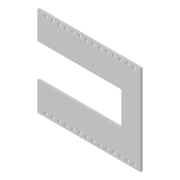
# Autodesk Inventor part: Flat Roof panel
Saved by Autodesk Inventor 2018 (Build 220112000, 112)
## iProperties
Created: 2019-01-04
Part Number: Flat Roof panel
Material: Generic
Document SubType Name: Modeling
Designer: ball
Density: 1 g/cm^3
Appearance: Default
Author: ball
Autodesk Inventor part; units mm, degrees
ref_plane "YZ Plane" through (0, 0, 0) normal (1, 0, 0) x (0, 1, 0)
ref_plane "XZ Plane" through (0, 0, 0) normal (0, 1, 0) x (-1, 0, 0)
ref_plane "Work Plane1" through (0, 0, 0) normal (0, 0, 1) x (1, 0, 0)
sketch "Sketch1" plane through (0, 0, 0) normal (0, 0, 1) x (1, 0, 0)
  line L0 (272, -4) -> (-8, -4) construction
  line L1 (230, 0) -> (230, -3.492) construction
  line L2 (272, 102.8084) -> (-8, 102.8084) construction
  line L3 (62, 0) -> (62, -4) construction
  line L4 (78, 0) -> (78, -3.492) construction
  circle A0 centre (220, 0) radius 2 construction
  circle A1 centre (164, 0) radius 2 construction
  circle A2 centre (148, 0) radius 2 construction
  circle A3 centre (140, 0) radius 2 construction
  circle A4 centre (132, 0) radius 2 construction
  circle A5 centre (124, 0) radius 2 construction
  circle A6 centre (116, 0) radius 2 construction
  circle A7 centre (116, 98.8084) radius 2 construction
  circle A8 centre (124, 98.8084) radius 2 construction
  circle A9 centre (132, 98.8084) radius 2 construction
  circle A10 centre (140, 98.8084) radius 2 construction
  circle A11 centre (148, 98.8084) radius 2 construction
  circle A12 centre (156, 98.8084) radius 2 construction
  circle A13 centre (164, 98.8084) radius 2 construction
  circle A14 centre (172, 98.8084) radius 2 construction
  circle A15 centre (180, 98.8084) radius 2 construction
  circle A16 centre (188, 98.8084) radius 2 construction
  circle A17 centre (196, 98.8084) radius 2 construction
  circle A18 centre (204, 98.8084) radius 2 construction
  circle A19 centre (212, 98.8084) radius 2 construction
  circle A20 centre (220, 98.8084) radius 2 construction
  circle A21 centre (212, 0) radius 2 construction
  circle A22 centre (204, 0) radius 2 construction
  circle A23 centre (196, 0) radius 2 construction
  circle A24 centre (188, 0) radius 2 construction
  circle A25 centre (180, 0) radius 2 construction
  circle A26 centre (172, 0) radius 2 construction
  circle A27 centre (156, 0) radius 2 construction
  circle A28 centre (220, 0) radius 2.2479
  circle A29 centre (211.999, 0) radius 2.2479
  circle A30 centre (203.998, 0) radius 2.2479
  circle A31 centre (195.997, 0) radius 2.2479
  circle A32 centre (187.996, 0) radius 2.2479
  circle A33 centre (179.995, 0) radius 2.2479
  circle A34 centre (171.994, 0) radius 2.2479
  circle A35 centre (163.993, 0) radius 2.2479
  circle A36 centre (155.992, 0) radius 2.2479
  circle A37 centre (147.991, 0) radius 2.2479
  circle A38 centre (139.99, 0) radius 2.2479
  circle A39 centre (131.989, 0) radius 2.2479
  circle A40 centre (123.988, 0) radius 2.2479
  circle A41 centre (115.987, 0) radius 2.2479
  circle A42 centre (220, 98.8084) radius 2.2479
  circle A43 centre (211.999, 98.8084) radius 2.2479
  circle A44 centre (203.998, 98.8084) radius 2.2479
  circle A45 centre (195.997, 98.8084) radius 2.2479
  circle A46 centre (187.996, 98.8084) radius 2.2479
  circle A47 centre (179.995, 98.8084) radius 2.2479
  circle A48 centre (171.994, 98.8084) radius 2.2479
  circle A49 centre (163.993, 98.8084) radius 2.2479
  circle A50 centre (155.992, 98.8084) radius 2.2479
  circle A51 centre (147.991, 98.8084) radius 2.2479
  circle A52 centre (139.99, 98.8084) radius 2.2479
  circle A53 centre (131.989, 98.8084) radius 2.2479
  circle A54 centre (123.988, 98.8084) radius 2.2479
  circle A55 centre (115.987, 98.8084) radius 2.2479
  line L5 (106.175, 30.29) -> (106.175, -3.492) construction
  line L6 (227.46, -3.492) -> (227.46, 102.3004) construction
  line L7 (106.175, 102.3004) -> (106.175, 69.6341) construction
  line L8 (205, 69.6341) -> (205, 30.29) construction
  line L9 (205, 69.6341) -> (205, 30.29) construction
  line L10 (106.175, 102.3004) -> (227.46, 102.3004)
  line L11 (227.46, 102.3004) -> (227.46, -3.492)
  line L12 (227.46, -3.492) -> (106.175, -3.492)
  line L13 (106.175, -3.492) -> (106.175, 30.29)
  line L14 (106.175, 30.29) -> (205, 30.29)
  line L15 (205, 30.29) -> (205, 69.6341)
  line L16 (205, 69.6341) -> (106.175, 69.6341)
  line L17 (106.175, 69.6341) -> (106.175, 102.3004)
  point P0 (0, 0)
  point P1 (-8, -4)
  dimension "d0" = 4.4958
  dimension "d3" = 8.001
  dimension "d8" = 4.4958
  dimension "d11" = 8.001
  constraints: 56 centre point, 34 end point, 13 equal radius, 13 horizontal alignment, 4 perpendicular, 3 vertical, 2 coincident, 2 collinear, 2 horizontal, 2 parallel, 94 other
  measures "d0" diameter of A28
  measures "d3" distance of A28.centre A29.centre
  measures "d8" diameter of A42
  measures "d11" distance of A42.centre A43.centre
extrude "Extrusion2" add sketch "Sketch1" along normal blind 2.54
body "Solid2"
